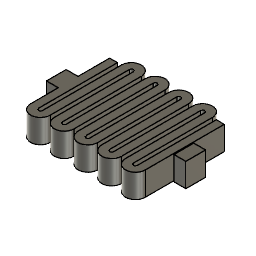
Spring (Autodesk Fusion 360 design; units mm, degrees)
part number: 2026-04-04-19-44-07-846
Autodesk Fusion 360 part; units mm, degrees
sketch "Sketch2" plane through (0, 0, 0) normal (0, 0, 1) x (1, 0, 0)
  line L0 (-0.5, 10) -> (-0.5, 0)
  line L1 (-1.5, 0) -> (-1.5, 10)
  line L2 (-2, 10) -> (-2, 0)
  line L3 (-3, 0) -> (-3, 10)
  arc A0 (-3, 0) -> (-0.5, 0) centre (-1.75, 0) ccw
  arc A1 (-2, 0) -> (-1.5, 0) centre (-1.75, 0) ccw
  arc A2 (0, 10) -> (-0.5, 10) centre (-0.25, 10) ccw
  arc A3 (1, 10) -> (-1.5, 10) centre (-0.25, 10) ccw
  line L4 (2.5, 10) -> (2.5, 0)
  line L5 (1.5, 0) -> (1.5, 10)
  line L6 (4, 0) -> (4, 10)
  line L7 (3, 10) -> (3, 0)
  line L8 (5.5, 10) -> (5.5, 0)
  line L9 (4.5, 0) -> (4.5, 10)
  arc A4 (1, 0) -> (1.5, 0) centre (1.25, 0) ccw
  arc A5 (3, 10) -> (2.5, 10) centre (2.75, 10) ccw
  arc A6 (4, 0) -> (4.5, 0) centre (4.25, 0) ccw
  arc A7 (0, 0) -> (2.5, 0) centre (1.25, 0) ccw
  arc A8 (4, 10) -> (1.5, 10) centre (2.75, 10) ccw
  arc A9 (3, 0) -> (5.5, 0) centre (4.25, 0) ccw
  line L10 (4.5, 10) -> (5.5, 10)
  line L11 (-4.5, 10) -> (-4.5, 0)
  line L12 (-3.5, 0) -> (-3.5, 10)
  line L13 (-6, 10) -> (-6, 0)
  line L14 (-5, 0) -> (-5, 10)
  arc A10 (-3, 10) -> (-3.5, 10) centre (-3.25, 10) ccw
  arc A11 (-2, 10) -> (-4.5, 10) centre (-3.25, 10) ccw
  arc A12 (-5, 0) -> (-4.5, 0) centre (-4.75, 0) ccw
  arc A13 (-6, 0) -> (-3.5, 0) centre (-4.75, 0) ccw
  line L15 (-7.5, 10) -> (-7.5, 0)
  line L16 (-6.5, 0) -> (-6.5, 10)
  line L17 (-9, 10) -> (-9, 0)
  line L18 (-8, 0) -> (-8, 10)
  arc A14 (-6, 10) -> (-6.5, 10) centre (-6.25, 10) ccw
  arc A15 (-5, 10) -> (-7.5, 10) centre (-6.25, 10) ccw
  arc A16 (-8, 0) -> (-7.5, 0) centre (-7.75, 0) ccw
  arc A17 (-9, 0) -> (-6.5, 0) centre (-7.75, 0) ccw
  line L19 (-9, 10) -> (-8, 10)
  line L20 (-10, 5) -> (-9, 5)
  line L21 (-9, 5) -> (-9, 3.5)
  line L22 (-9, 3.5) -> (-10, 3.5)
  line L23 (-10, 3.5) -> (-10, 5)
  line L24 (5.5, 5) -> (6.5, 5)
  line L25 (6.5, 5) -> (6.5, 3.5)
  line L26 (6.5, 3.5) -> (5.5, 3.5)
  line L27 (5.5, 3.5) -> (5.5, 5)
  line L28 (0, 10) -> (0, 0)
  line L29 (1, 0) -> (1, 10)
  constraint vertical L0
  constraint vertical L1
  constraint vertical L2
  constraint vertical L3
  constraint tangent L0 A0
  constraint tangent L3 A0
  constraint tangent L1 A1
  constraint tangent L2 A1
  constraint tangent L0 A2
  constraint tangent L1 A3
  constraint vertical L4
  constraint vertical L5
  constraint vertical L6
  constraint vertical L7
  constraint vertical L8
  constraint vertical L9
  constraint tangent L5 A4
  constraint tangent L7 A5
  constraint tangent L4 A5
  constraint tangent L9 A6
  constraint tangent L6 A6
  constraint tangent L4 A7
  constraint coincident A7.start L28.end
  constraint tangent L6 A8
  constraint tangent L5 A8
  constraint tangent L8 A9
  constraint tangent L7 A9
  constraint perpendicular L8 L10
  constraint vertical L11
  constraint vertical L12
  constraint vertical L13
  constraint vertical L14
  constraint tangent L3 A10
  constraint tangent L12 A10
  constraint tangent L11 A11
  constraint tangent L2 A11
  constraint tangent L14 A12
  constraint tangent L13 A13
  constraint tangent L12 A13
  constraint vertical L15
  constraint vertical L16
  constraint vertical L17
  constraint vertical L18
  constraint tangent L13 A14
  constraint tangent L16 A14
  constraint tangent L14 A15
  constraint tangent L15 A15
  constraint tangent L15 A16
  constraint tangent L17 A17
  constraint tangent L16 A17
  constraint perpendicular L18 L19
  constraint horizontal L20
  constraint vertical L21
  constraint horizontal L22
  constraint vertical L23
  constraint coincident L17 L21.end
  constraint horizontal L24
  constraint vertical L25
  constraint horizontal L26
  constraint vertical L27
  constraint midpoint L8 L24.start
  constraint tangent A7 L28
  constraint tangent A3 L29
extrude "Extrude1" add sketch "Sketch2" along normal blind 3 contours L0 L1 L2 L3 A0 A1 A2 A3 L4 L5 L6 L7 L8 L9 A4 A5 A6 A7 A8 A9 L10 L11 L12 L13 L14 A10 A11 A12 A13 L15 L16 L17 L18 A14 A15 A16 A17 L19 L21 L27 L28 L29 makes body 1
sketch "Sketch3" plane through (0, 0, 0) normal (0, 0, 1) x (1, 0, 0)
  line L0 (-10.5, 6) -> (-9, 6)
  line L1 (-9, 6) -> (-9, 3.5)
  line L2 (-9, 3.5) -> (-10.5, 3.5)
  line L3 (-10.5, 3.5) -> (-10.5, 6)
  line L4 (5.6259, 6) -> (7.1259, 6)
  line L5 (7.1259, 6) -> (7.1259, 3.5)
  line L6 (7.1259, 3.5) -> (5.6259, 3.5)
  line L7 (5.6259, 3.5) -> (5.6259, 6)
  dimension "d5" = 1.5
  constraint horizontal L0
  constraint vertical L1
  constraint horizontal L2
  constraint vertical L3
  constraint horizontal L4
  constraint vertical L5
  constraint horizontal L6
  constraint vertical L7
  measures "d5" distance of L4.start L4.end
extrude "Extrude2" add sketch "Sketch3" along normal blind 3 bodies 1 makes body 2 at (7.1259, 5.1667, 1)
